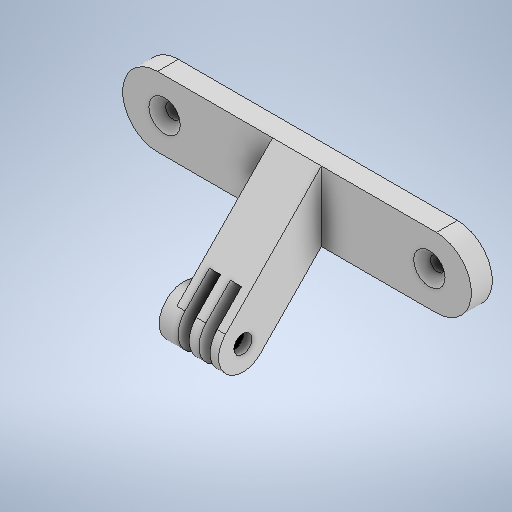
# Autodesk Inventor part: support_gopro
Saved by Autodesk Inventor 2025.2 (Build 292293000, 293)
## iProperties
Created: 2025-05-12
Part Number: support_gopro
Material: Générique
Document SubType Name: Modeling
Designer: enezl
Density: 1 g/cm^3
Appearance: Par défaut
Author: enezl
Autodesk Inventor part; units mm, degrees
ref_plane "YZ Plane" through (0, 0, 0) normal (1, 0, 0) x (0, 1, 0)
ref_plane "XZ Plane" through (0, 0, 0) normal (0, 1, 0) x (-1, 0, 0)
ref_plane "XY Plane" through (0, 0, 0) normal (0, 0, 1) x (1, 0, 0)
sketch "Esquisse1" plane through (0, 0, 0) normal (0, 0, 1) x (1, 0, 0)
  line L0 (-40, 0) -> (40, 0) construction
  line L1 (-40, -10) -> (40, -10)
  line L2 (40, 10) -> (-40, 10)
  arc A0 (-40, 10) -> (-40, -10) centre (-40, 0) ccw
  arc A1 (40, -10) -> (40, 10) centre (40, 0) ccw
  point P0 (0, 0)
  point P1 (0, 0)
  dimension "d0" = 20
  dimension "d1" = 80
  constraints: 8 end point, 4 point on circle, 4 tangent, 3 coincident, 2 centre point, 1 horizontal, 1 midpoint, 1 parallel
  measures "d0" distance between parallel lines of L1 L2
  measures "d1" distance of L0.start L0.end
extrude "Extrusion1" add sketch "Esquisse1" along normal blind 6
sketch "Esquisse2" plane through (0, 0, 6) normal (0, 0, 1) x (1, 0, 0)
  line L0 (-37.9704, 0) -> (37.9704, 0) construction
  point P0 (0, 0)
  point P1 (0, 0)
  constraints: 2 end point, 1 coincident, 1 horizontal, 1 midpoint
hole "Perçage1" at (-37.9704, 0, 6) at (37.9704, 0, 6) direction (0, 0, -1) diameter 4.2 depth 6 countersink diameter 9 countersink angle 90
sketch "Esquisse3" plane through (0, 0, 0) normal (1, 0, 0) x (0, 1, 0)
  line L0 (10, 6) -> (-10, 6) projected
  line L1 (10, 6) -> (-18.0536, 33.498)
  line L2 (-10, 0) -> (-10, 6) projected
  line L3 (-10, 6) -> (-27.8536, 23.5)
  arc A0 (-18.0536, 33.498) -> (-27.8536, 23.5) centre (-22.9536, 28.499) ccw
  circle A1 centre (-22.9536, 28.499) radius 2.6
  point P0 (0, 0)
  dimension "d11" = 14
  dimension "d12" = 5.2
  dimension "d13" = 25
  constraints: 4 end point, 2 centre point, 2 point on circle, 2 tangent, 1 coincident, 1 parallel
  measures "d11" distance between parallel lines of L3 L1
  measures "d12" diameter of A1
  measures "d13" distance of L0.end L3.end
extrude "Extrusion2" add sketch "Esquisse3" along normal mid plane 14
sketch "Esquisse4" plane through (-7, -18.0536, 33.498) normal (0, 0.7, 0.7141) x (1, 0, 0)
  line L0 (11.6, -10) -> (8.4, -10)
  line L1 (8.4, -10) -> (8.4, 10)
  line L2 (8.4, 10) -> (11.6, 10)
  line L3 (11.6, 10) -> (11.6, -10)
  line L4 (0, 0) -> (14, 0) projected
  line L5 (11.6, -10) -> (8.4, 10) construction
  line L6 (8.4, -10) -> (11.6, 10) construction
  line L7 (7, 0) -> (7, 13.553)
  line L8 (2.4, -10) -> (5.6, -10)
  line L9 (5.6, -10) -> (5.6, 10)
  line L10 (5.6, 10) -> (2.4, 10)
  line L11 (2.4, 10) -> (2.4, -10)
  line L12 (2.4, -10) -> (5.6, 10) construction
  line L13 (5.6, -10) -> (2.4, 10) construction
  point P0 (7, 36.3414)
  point P1 (10, 0)
  point P2 (4, 0)
  dimension "d16" = 3.2
  dimension "d17" = 20
  dimension "d18" = 1.4
  constraints: 26 end point, 5 symmetric about line, 3 midpoint, 2 parallel, 1 horizontal, 1 perpendicular, 1 point on line, 1 vertical
  measures "d16" distance of L1.end L2.end
  measures "d17" distance of L2.end L0.start
  measures "d18" distance from line of L7.start L1
extrude "Extrusion3" cut sketch "Esquisse4" along normal through all both and the other way through all
sketch "Esquisse5" plane through (-7, 0, 0) normal (-1, 0, 0) x (0, 0, 1)
  circle A0 centre (28.499, -22.9536) radius 2.6 construction
  circle A1 centre (28.499, -22.9536) radius 7
  line L0 (33.498, -18.0536) -> (6, 10) construction
  line L1 (28.499, -18.3348) -> (32.499, -20.6442)
  line L2 (32.499, -20.6442) -> (32.499, -25.263)
  line L3 (32.499, -25.263) -> (28.499, -27.5724)
  line L4 (28.499, -27.5724) -> (24.499, -25.263)
  line L5 (24.499, -25.263) -> (24.499, -20.6442)
  line L6 (24.499, -20.6442) -> (28.499, -18.3348)
  line L7 (28.499, -22.9536) -> (28.499, -18.3348) construction
  point P0 (0, 0)
  dimension "d21" = 8
  constraints: 14 end point, 2 coincident, 1 vertical, 16 other
  measures "d21" distance between parallel lines of L2 L5
extrude "Extrusion4" add sketch "Esquisse5" along normal blind 3
